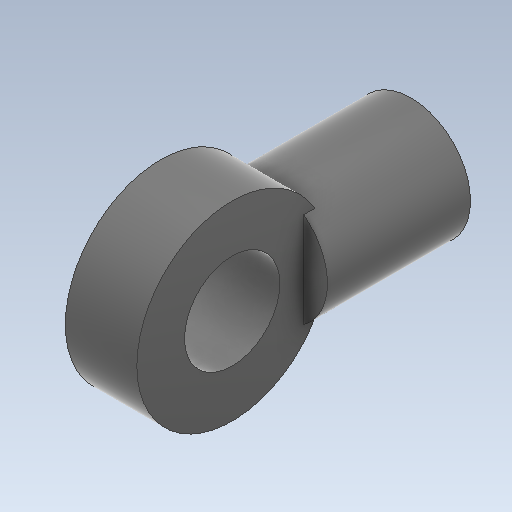
# Autodesk Inventor part: 尻
Saved by Autodesk Inventor 2020 (Build 240168000, 168)
## iProperties
Created: 2020-03-29
Part Number: 尻
Material: ABS プラスチック
Document SubType Name: Modeling
Designer: happy
Density: 1.06 g/cm^3
Appearance: 滑らか - 黒
Author: happy
Autodesk Inventor part; units mm, degrees
ref_plane "YZ Plane" through (0, 0, 0) normal (1, 0, 0) x (0, 1, 0)
ref_plane "XZ Plane" through (0, 0, 0) normal (0, 1, 0) x (-1, 0, 0)
ref_plane "XY Plane" through (0, 0, 0) normal (0, 0, 1) x (1, 0, 0)
sketch "スケッチ1" plane through (0, 0, 0) normal (0, 0, 1) x (1, 0, 0)
  circle A0 centre (0, 0) radius 2.5
  dimension "d0" = 5
  constraints: 1 centre point, 1 coincident
  measures "d0" diameter of A0
extrude "押し出し1" add sketch "スケッチ1" along normal blind 5
sketch "スケッチ2" plane through (0, 0, 0) normal (1, 0, 0) x (0, 1, 0)
  line L0 (2.5, 5) -> (-2.5, 5) projected
  line L1 (2.5, 0) -> (-2.5, 0) projected
  circle A0 centre (0, 9) radius 2
  circle A1 centre (0, 9) radius 4
  line L2 (2.5, 5) -> (-2.5, 5) projected
  point P0 (0, 0)
  dimension "d3" = 4
  dimension "d4" = 8
  constraints: 2 centre point, 1 coincident, 1 tangent
  measures "d3" diameter of A0
  measures "d4" diameter of A1
sketch "スケッチ3" plane through (0, 0, 5) normal (0, 0, 1) x (1, 0, 0)
  circle A0 centre (0, 0) radius 2.5 projected
extrude "押し出し2" add sketch "スケッチ3" along normal blind 1
extrude "押し出し3" add sketch "スケッチ2" along normal mid plane 3
